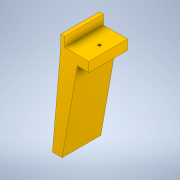
# Autodesk Inventor part: Leg-01
Saved by Autodesk Inventor 2022 (Build 260153000, 153)
## iProperties
Created: 2023-05-22
Part Number: Leg-01
Material: Aluminum 6061
Document SubType Name: Modeling
Designer: brenden_deutschman
Density: 2.7 g/cm^3
Appearance: Aluminum - Flat
Mass: 352.083 g
Surface Area: 228.346 cm^2
Volume: 130.401 cm^3
Description: Aluminum 5 Inch Tall Leg
Author: brenden_deutschman
Title: Leg
Autodesk Inventor part; units mm, degrees
ref_plane "YZ Plane" through (0, 0, 0) normal (1, 0, 0) x (0, 1, 0)
ref_plane "XZ Plane" through (0, 0, 0) normal (0, 1, 0) x (-1, 0, 0)
ref_plane "XY Plane" through (0, 0, 0) normal (0, 0, 1) x (1, 0, 0)
sketch "Sketch1" plane through (0, 0, 0) normal (0, 0, 1) x (1, 0, 0)
  line L0 (0, 0) -> (-6.35, 0)
  line L1 (-6.35, 0) -> (4.7611, 127)
  line L2 (0, 0) -> (6.35, 0)
  line L3 (6.35, 0) -> (82.55, 0) construction
  line L4 (6.35, 0) -> (28.7435, 127)
  line L5 (6.35, 0) -> (135.3092, 0) construction
  line L6 (28.7435, 127) -> (4.7611, 127)
  dimension "d0" = 6.35
  dimension "d2" = 85
  dimension "d3" = 6.35
  dimension "d6" = 80
  dimension "d9" = 127
  constraints: 14 end point, 4 horizontal, 1 equal length, 1 point on line
  measures "d0" distance of L0.start L0.end
  measures "d2" angle of L0 L1
  measures "d3" distance of L0.start L2.end
  measures "d6" angle of L5 L4
  measures "d9" distance between parallel lines of L0 L6
extrude "Extrusion1" add sketch "Sketch1" along normal blind 50.8
sketch "Sketch2" plane through (4.7611, 127, 0) normal (0, 1, 0) x (1, 0, 0)
  line L0 (0, 0) -> (-11.1111, 0) projected
  line L1 (0, 0) -> (5.08, 0)
  line L2 (23.9825, 0) -> (0, 0) projected
  line L3 (5.08, 0) -> (5.08, -50.8)
  line L4 (23.9825, -50.8) -> (0, -50.8) projected
  line L5 (0, 0) -> (0, -50.8) projected
  line L6 (0, -50.8) -> (0, 0)
  point P0 (-4.7611, 0)
  dimension "d10" = 5.08
  constraints: 6 end point, 2 point on line, 1 perpendicular, 1 vertical
  measures "d10" distance of L0.start L1.end
extrude "Extrusion2" add sketch "Sketch2" along normal blind 12.7
sketch "Sketch4" plane through (28.7435, 127, 50.8) normal (0, 1, 0) x (1, 0, 0)
  line L0 (0, 50.8) -> (-18.9025, 50.8) projected
  line L1 (0, 50.8) -> (12.7, 50.8)
  line L2 (12.7, 50.8) -> (12.7, 0)
  line L3 (0, 50.8) -> (0, 0) projected
  line L4 (12.7, 0) -> (0, 0)
  line L5 (-18.9025, 0) -> (-18.9025, 50.8) projected
  line L6 (0, 0) -> (-18.9025, 0)
  line L7 (-18.9025, 0) -> (-18.9025, 50.8)
  line L8 (-18.9025, 50.8) -> (0, 50.8)
  point P0 (-28.7435, 50.8)
  dimension "d14" = 12.7
  constraints: 12 end point, 3 perpendicular, 1 collinear, 1 horizontal, 1 parallel
  measures "d14" distance of L0.start L1.end
extrude "Extrusion3" add sketch "Sketch4" against normal blind 12.7
sketch "Sketch5" plane through (9.8411, 127, 50.8) normal (0, 1, 0) x (1, 0, 0)
  line L0 (31.6025, 0) -> (31.6025, 50.8) projected
  line L1 (16.6631, 50.8) -> (16.6631, 0) projected
  circle A0 centre (20.1725, 25.4) radius 1.7526
  line L2 (31.6025, 50.8) -> (0, 50.8) projected
  point P0 (-9.8411, 50.8)
  dimension "d18" = 3.5052
  dimension "d19" = 11.43
  dimension "d20" = 25.4
  constraints: 1 centre point
  measures "d18" diameter of A0
  measures "d19" distance from line of L0 A0.centre
  measures "d20" distance from line of L2 A0.centre
extrude "Extrusion4" cut sketch "Sketch5" against normal blind 12.7
thread "Thread1" size "6-32 UNC" class "2B" standard "ANSI Unified Screw Threads" full length
body "Solid1"
